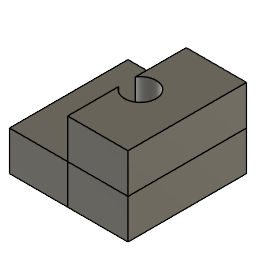
New assembly (Autodesk Fusion 360 archive; units mm, degrees)
design "Z smooth rod holder"
part number: 2025-12-29-13-48-08-419
Autodesk Fusion 360 part; units mm, degrees
sketch "Sketch1" plane through (0, 0, 0) normal (0, 0, 1) x (1, 0, 0)
  line L0 (0, 0) -> (30, 0)
  line L1 (30, 0) -> (30, 30)
  line L2 (30, 30) -> (0, 30)
  line L3 (0, 30) -> (0, 0)
  circle A0 centre (13, 15) radius 2.75
  circle A1 centre (18.14, 15) radius 4
  line L4 (14.7492, 17.122) -> (14.7492, 12.878)
  line L5 (14.7492, 12.878) -> (14.7492, 0)
  line L6 (14.7492, 0) -> (14.7492, 30)
  dimension "d1" = 30
  dimension "d2" = 30
  dimension "d3" = 5.5
  dimension "d4" = 13
  dimension "d5" = 8
  dimension "d6" = 15
  dimension "d7" = 15
  dimension "d8" = 5.14
  constraint horizontal L0
  constraint vertical L1
  constraint horizontal L2
  constraint vertical L3
  constraint coincident L0.start L3.end
  constraint coincident A1 L4.start
  constraint coincident A0 L4.start
  constraint coincident A1 L4.end
  constraint coincident A0 L4.end
  constraint coincident L0 L5.end
  constraint perpendicular L0 L5
  constraint coincident L2 L6.end
  constraint perpendicular L2 L6
  measures "d1" distance of L1 L3
  measures "d2" distance of L0 L2
  measures "d3" diameter of A0
  measures "d4" distance of L3 A0.centre
  measures "d5" diameter of A1
  measures "d6" distance of L0 A0.centre
  measures "d7" distance of L0 A1.centre
  measures "d8" distance of A0.centre A1.centre
extrude "Extrude1" add sketch "Sketch1" along normal blind 10 contours L0 L2 L3 A0 L5 L6 | L0 L1 L2 A1 L5 L6 makes body 1
extrude "Extrude2" add sketch "Sketch1" along normal blind 20 separate body contours L0 L1 L2 A1 L5 L6 makes body 2

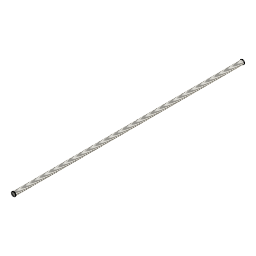
design "420mm t8 leadscrew"
part number: 2026-02-08-12-54-06-980
Autodesk Fusion 360 part; units mm, degrees
sketch "Sketch1" plane through (0, 0, 0) normal (0, 1, 0) x (1, 0, 0)
  circle A0 centre (0, 0) radius 4
  dimension "d1" = 8
  constraint coincident A0.centre origin
  measures "d1" diameter of A0
extrude "Extrude1" add sketch "Sketch1" along normal blind 420
thread "Thread1" "ISO Metric profile 8.0 M8x1.25 M8x1.25 6g" major diameter 7.866 minor diameter 6.4455 pitch 1.25 angle 60 resizes the face on face at (-1.7535, 280, 3.5952)

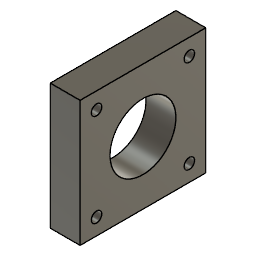
design "Nema 17 face mount"
part number: 2025-12-27-18-46-16-654
Autodesk Fusion 360 part; units mm, degrees
sketch "Sketch1" plane through (0, 0, 0) normal (1, 0, 0) x (0, 1, 0)
  line L0 (5, 30) -> (25, 30)
  line L1 (25, 30) -> (25, 0)
  line L2 (25, 0) -> (5, 0)
  line L3 (5, 0) -> (5, 30)
  circle A0 centre (15, 15) radius 4
  dimension "d1" = 8
  dimension "d2" = 10
  dimension "d3" = 20
  dimension "d4" = 15
  dimension "d5" = 15
  dimension "d6" = 30
  constraint horizontal L0
  constraint vertical L1
  constraint horizontal L2
  constraint vertical L3
  measures "d1" diameter of A0
  measures "d2" distance of L1 A0.centre
  measures "d3" distance of L1 L3
  measures "d4" distance of L2 A0.centre
  measures "d5" distance of L0 A0.centre
  measures "d6" distance of L0 L2
sketch "Sketch2" plane through (0, 0, 0) normal (1, 0, 0) x (0, 1, 0)
  line L0 (0, 0) -> (42, 0)
  line L1 (42, 0) -> (42, 42)
  line L2 (42, 42) -> (0, 42)
  line L3 (0, 42) -> (0, 0)
  circle A0 centre (21, 21) radius 11
  circle A1 centre (5.5, 36.5) radius 1.75
  circle A2 centre (36.5, 36.5) radius 1.75
  circle A3 centre (5.5, 5.5) radius 1.75
  circle A4 centre (36.5, 5.5) radius 1.75
  dimension "d9" = 42
  dimension "d10" = 42
  dimension "d11" = 22
  dimension "d12" = 3.5
  dimension "d13" = 3.5
  dimension "d14" = 3.5
  dimension "d15" = 3.5
  dimension "d16" = 5.5
  dimension "d17" = 5.5
  dimension "d18" = 5.5
  dimension "d19" = 5.5
  dimension "d20" = 5.5
  dimension "d21" = 5.5
  dimension "d22" = 5.5
  dimension "d23" = 5.5
  dimension "d24" = 21
  dimension "d25" = 21
  constraint horizontal L0
  constraint vertical L1
  constraint horizontal L2
  constraint vertical L3
  constraint coincident L0.start L3.end
  measures "d9" distance of L0.start L2.end
  measures "d10" distance of L1 L3
  measures "d11" diameter of A0
  measures "d12" diameter of A1
  measures "d13" diameter of A2
  measures "d14" diameter of A3
  measures "d15" diameter of A4
  measures "d16" distance of L1 A2.centre
  measures "d17" distance of L2 A2.centre
  measures "d18" distance of L2 A1.centre
  measures "d19" distance of L3 A1.centre
  measures "d20" distance of L3 A3.centre
  measures "d21" distance of L0 A3.centre
  measures "d22" distance of L0 A4.centre
  measures "d23" distance of L1 A4.centre
  measures "d24" distance of L3 A0.centre
  measures "d25" distance of L0 A0.centre
extrude "Extrude2" add sketch "Sketch2" along normal blind 10

design "Hexagon Regular Nut DIN EN ISO 4032 - M5 Steel 6 Plain"
description: Hexagon Regular Nut DIN EN ISO 4032 - M5
part number: DIN EN ISO 4032 - M5 Steel 6 Plain
Autodesk Fusion 360 part; units mm, degrees
sketch "Sketch1" plane through (0, 0, 0) normal (0, 1, 0) x (1, 0, 0)
  line L0 (0, 0) -> (0, -4.7)
  line L1 (-2.5, 0) -> (-3.92, 0)
  line L2 (-3.92, 0) -> (-4.62, -0.4041)
  line L3 (-4.62, -0.4041) -> (-4.62, -4.2959)
  line L4 (-4.62, -4.2959) -> (-3.92, -4.7)
  line L5 (-3.92, -4.7) -> (-2.5, -4.7)
  line L6 (-2.5, -4.7) -> (-2.5, 0)
  dimension "d121" = 5
  dimension "d122" = 30
  dimension "d123" = 30
  dimension "d128" = 9.24
  dimension "d172" = 7.84
  dimension "d179" = 4.7
  constraint vertical L0
  constraint coincident L0 L0.end
  constraint coincident origin L0
  constraint horizontal L1
  constraint coincident L0.start L1
  constraint coincident L0.start origin
  constraint coincident L0.end L5
  constraint vertical L1.end L4.end
  measures "d122" angle of L1 L2
  measures "d123" angle of L4 L5
  measures "d179" distance of L1 L5
revolve "Revolve1" add sketch "Sketch1" angle 360 about axis through (0, 0, 0) along (0, 0, 1)
sketch "Sketch8" plane through (0, 0, 4.7) normal (0, 0, 1) x (1, 0, 0)
  line L0 (-4, -2.3118) -> (-4, 2.3118)
  circle A0 centre (0, 0) radius 2.5
  circle A1 centre (0, 0) radius 4.62
  dimension "d114" = 4
  constraint coincident L0.end A1
  constraint coincident L0.start A1
  constraint vertical L0
  measures "d114" distance of A0.centre L0
extrude "Extrude5" cut sketch "Sketch8" against normal blind 4.7 contours L0 A1 picked at (-4.1, -0.5631)
pattern_circular "C-Pattern2" count 6 over 360 about axis through (0, 0, 1.75) along (0, 0, 1) of "Extrude5"
thread "Thread3" "ISO Metric profile 5.0 M5x0.8 M5x0.8 6H" major diameter 5.12 minor diameter 4.234 pitch 0.8 angle 60 resizes the face on face at (-2.4876, 0.2489, 3.1333)
sketch "Sketch12" plane through (0, 0, 0) normal (0, 1, 0) x (1, 0, 0)
  line L0 (-2.5, 0) -> (0, 0)
  line L1 (-1.1432, -2.35) -> (-2.5, 0)
  line L2 (-2.5, -4.7) -> (0, -4.7)
  line L3 (-1.1432, -2.35) -> (-2.5, -4.7)
  line L4 (0, 0) -> (0, -4.7)
  dimension "d169" = 60
  dimension "d177" = 2.5
  dimension "d178" = 60
  constraint horizontal L0
  constraint coincident L1.start L3.start
  constraint vertical L0.start L2.start
  constraint coincident L2.end L4.end
  constraint coincident L0.end L4.start
  constraint perpendicular L2 L4
  measures "d169" angle of L2 L3
  measures "d177" distance of L0.start L4
  measures "d178" angle of L0 L1
revolve "Revolve3" cut sketch "Sketch12" angle 360 about axis through (0, 0, 1.75) along (0, 0, 1)
equation "adsk_nheig = 4.70 mm"
equation "adsk_maxdia = 9.24 mm"
equation "adsk_nomdia = 5.00 mm"
equation "d89 = -adsk_nheig"
equation "adsk_waflat = 8.00 mm"
equation "d114 = adsk_waflat / 2"
equation "adsk_chamang1 = 30.00 deg"
equation "adsk_chamang2 = 30.00 deg"
equation "d121 = adsk_nomdia"
equation "d122 = adsk_chamang1"
equation "d123 = adsk_chamang2"
equation "d128 = adsk_maxdia"
equation "d163 = adsk_nheig"
equation "adsk_beardia = 7.84 mm"
equation "d172 = adsk_beardia"
equation "d177 = adsk_nomdia * 0.5"
equation "d179 = adsk_nheig"

design "GT2 Idle pulley"
part number: 2025-12-12-13-43-18-296
Autodesk Fusion 360 part; units mm, degrees
sketch "Sketch1" plane through (0, 0, 0) normal (0, 1, 0) x (1, 0, 0)
sketch "Sketch2" plane through (0, 0, 0) normal (0, 1, 0) x (1, 0, 0)
  circle A0 centre (0, 0) radius 7
  circle A1 centre (0, 0) radius 9
  circle A2 centre (0, 0) radius 2.5
  dimension "d11" = 14
  dimension "d12" = 18
  dimension "d13" = 5
  constraint coincident A0.centre A1.centre
  constraint concentric A0 A1
  constraint concentric A0 A2
  measures "d11" diameter of A0
  measures "d12" diameter of A1
  measures "d13" diameter of A2
extrude "Extrude4" add sketch "Sketch2" along normal blind 1 contours A0 | A1
extrude "Extrude5" add sketch "Sketch2" along normal blind 7.5 contours A0
extrude "Extrude6" add sketch "Sketch2" along normal blind 1 from surface at 7.5 contours A1

design "Hex Head Bolt JIS B 1180 - M5x40 - C Steel 4.6 Plain"
description: Hex Head Bolt JIS B 1180 - M5x40 - C
part number: JIS B 1180 - M5x40 C Steel 4.6 Plain
Autodesk Fusion 360 part; units mm, degrees
sketch "Sketch1" plane through (0, 0, 0) normal (0, 1, 0) x (1, 0, 0)
  line L0 (-2.5, 0) -> (-2.5, 40)
  line L1 (-2.5, 40) -> (0, 40)
  line L2 (0, 40) -> (0, -3.5)
  line L3 (-2.5, 0) -> (-4.5712, 0)
  line L4 (-4.5712, 0) -> (-4.5712, -3.124)
  line L5 (-3.92, -3.5) -> (0, -3.5)
  line L6 (-4.5712, -3.124) -> (-3.92, -3.5)
  dimension "d81" = 9.1424
  dimension "d135" = 5
  dimension "d139" = 3.5
  dimension "d140" = 40
  dimension "d156" = 7.84
  dimension "d158" = 30
  constraint perpendicular L0 L1
  constraint collinear origin L1.end L2.end
  constraint perpendicular L0 L3
  constraint coincident origin L3
  constraint vertical L2
  constraint coincident L2 L5.end
  constraint coincident L0.start L3.start
  constraint coincident L0.end L1.start
  constraint vertical L4
  measures "d139" distance of L3 L5
  measures "d140" distance of L1 L3
  measures "d158" angle of L5 L6
revolve "Revolve1" add sketch "Sketch1" angle 360 about axis through (0, 0, -40) along (0, 0, 1)
sketch "Sketch8" plane through (0, 0, 3.5) normal (0, 0, 1) x (1, 0, 0)
  circle A0 centre (0, 0) radius 4.5712
  line L0 (-3.9588, -2.2856) -> (0, -4.5712)
  line L1 (0, -4.5712) -> (3.9588, -2.2856)
  line L2 (3.9588, -2.2856) -> (3.9588, 2.2856)
  line L3 (3.9588, 2.2856) -> (0, 4.5712)
  line L4 (0, 4.5712) -> (-3.9588, 2.2856)
  line L5 (-3.9588, 2.2856) -> (-3.9588, -2.2856)
  constraint coincident A0 L0.start
  constraint coincident A0.centre origin
  constraint vertical L5
extrude "Extrude5" cut sketch "Sketch8" against normal blind 3.5 contours A0 L2 | A0 L3 | A0 L1 | A0 L4 | A0 L0 | A0 L5
fillet "Fillet7" radius 0.2 1 edges at (-2.3308, 0.904, 0)
thread "Thread4" "ISO Metric profile 5.0 M5x0.8 M5x0.8 6g" major diameter 4.901 minor diameter 3.9895 pitch 0.8 angle 60 resizes the face on face at (-2.4969, 0.1246, -13.4667) from (0, 0, -1.6) to (0, 0, -40)
sketch "Sketch13" plane through (0, 0, 0) normal (0, 1, 0) x (1, 0, 0)
  line L0 (0, 40) -> (0, -3.5) construction
  line L1 (0, 40) -> (-2.55, 40)
  line L2 (-2.55, 40) -> (-2.55, 39.5)
  line L3 (-2.55, 39.5) -> (-2, 40)
  dimension "d160" = 0.5
  dimension "d161" = 2
  dimension "d162" = 2.55
  constraint coincident L0.start L1.start
  constraint perpendicular L0 L1
  constraint perpendicular L1 L2
  constraint coincident L1 L3.end
  measures "d160" distance of L1 L2.end
  measures "d161" distance of L0 L3.end
  measures "d162" distance of L0.start L2
revolve "Revolve4" cut sketch "Sketch13" angle 360 about axis through (0, 0, 1.75) along (0, 0, 1)
equation "adsk_nomlen = 40.00 mm"
equation "adsk_headh = 3.50 mm"
equation "adsk_headdia = 9.1424 mm"
equation "adsk_nomdia = 5.00 mm"
equation "d81 = adsk_headdia"
equation "d89 = -adsk_headh"
equation "adsk_waflat = 8.00 mm"
equation "adsk_thrlen = 38.40 mm"
equation "adsk_midfillet = 0.20 mm"
equation "d135 = adsk_nomdia"
equation "d139 = adsk_headh"
equation "d140 = adsk_nomlen"
equation "d142 = adsk_midfillet"
equation "adsk_endpointdia = adsk_nomdia - adsk_startlen * 2"
equation "adsk_startlen = 0.1 * adsk_nomdia"
equation "d156 = adsk_waflat * 0.98"
equation "d158 = adsk_chamang2"
equation "adsk_chamang2 = 30.00 deg"
equation "d160 = adsk_startlen"
equation "d161 = adsk_endpointdia / 2"
equation "d162 = adsk_nomdia * 0.51"
equation "d166 = min(adsk_thrlen; adsk_nomlen - adsk_midfillet - 0.001 mm)"

design "500mm smooth rod"
part number: 2026-02-07-13-03-38-961
Autodesk Fusion 360 part; units mm, degrees
sketch "Sketch1" plane through (0, 0, 0) normal (0, 1, 0) x (1, 0, 0)
  circle A0 centre (0, 0) radius 4
  dimension "d1" = 8
  constraint coincident A0.centre origin
  measures "d1" diameter of A0
extrude "Extrude1" add sketch "Sketch1" along normal blind 500
extrude "Extrude2" cut 1 faces at (1.4202, 500, 0.5286) along direction (0, -1, 0) blind 15
